Autodesk Fusion 360 part; units mm, degrees
(part 2 of 2)
sketch "Sketch9" plane through (0, 0, 0) normal (1, 0, 0) x (0, 1, 0)
  line L0 (195.5, 133.4393) -> (195.5, 130.2075)
  line L1 (208.5, 133) -> (208.5, 135.95)
  line L2 (196.5607, 125.5) -> (199.7925, 125.5)
  line L3 (190, 133.5) -> (190, 138.5)
  line L4 (190.5, 133) -> (190.5, 133.5)
  line L5 (205.95, 138.5) -> (205.95, 137.0107)
  line L6 (203.5, 140) -> (208.5, 140)
  line L7 (190, 126.5) -> (190.5, 126.5)
  line L8 (203.4393, 125.5) -> (200.2075, 125.5)
  line L9 (210, 126.5) -> (209.5, 126.5)
  line L10 (203.5, 120) -> (203.5, 120.5)
  line L11 (208.5, 124.05) -> (207.0107, 124.05)
  line L12 (192.9893, 124.05) -> (195.5, 126.5607)
  line L13 (190, 121.5) -> (190, 126.5)
  line L14 (209.5, 127) -> (208.5, 127)
  line L15 (194.05, 121.5) -> (194.05, 122.9893)
  line L16 (205.95, 137.0107) -> (203.4393, 134.5)
  line L17 (194.05, 138.5) -> (194.05, 137.0107)
  line L18 (191.5, 135.95) -> (192.9893, 135.95)
  line L19 (205.95, 121.5) -> (205.95, 122.9893)
  line L20 (197, 121.5) -> (194.05, 121.5)
  line L21 (209.5, 133.5) -> (209.5, 133)
  line L22 (209.5, 127) -> (209.5, 126.5)
  line L23 (208.5, 127) -> (208.5, 124.05)
  line L24 (197, 139.5) -> (197, 138.5)
  line L25 (203, 120.5) -> (203, 121.5)
  line L26 (196.5, 120) -> (191.5, 120)
  line L27 (196.5, 139.5) -> (197, 139.5)
  line L28 (210, 126.5) -> (210, 121.5)
  line L29 (204.5, 126.5607) -> (204.5, 129.7925)
  line L30 (205.95, 122.9893) -> (203.4393, 125.5)
  line L31 (208.5, 135.95) -> (207.0107, 135.95)
  line L32 (195.5, 126.5607) -> (195.5, 129.7925)
  line L33 (197, 120.5) -> (196.5, 120.5)
  line L34 (196.5, 140) -> (196.5, 139.5)
  line L35 (203, 139.5) -> (203.5, 139.5)
  line L36 (194.05, 137.0107) -> (196.5607, 134.5)
  line L37 (203, 139.5) -> (203, 138.5)
  line L38 (207.0107, 124.05) -> (204.5, 126.5607)
  line L39 (190, 133.5) -> (190.5, 133.5)
  line L40 (191.5, 140) -> (196.5, 140)
  line L41 (191.5, 127) -> (191.5, 124.05)
  line L42 (191.5, 124.05) -> (192.9893, 124.05)
  line L43 (203, 121.5) -> (205.95, 121.5)
  line L44 (190.5, 126.5) -> (190.5, 127)
  line L45 (196.5607, 134.5) -> (199.7925, 134.5)
  line L46 (203.5, 120.5) -> (203, 120.5)
  line L47 (203, 138.5) -> (205.95, 138.5)
  line L48 (192.9893, 135.95) -> (195.5, 133.4393)
  line L49 (203.5, 140) -> (203.5, 139.5)
  line L50 (210, 133.5) -> (209.5, 133.5)
  line L51 (197, 120.5) -> (197, 121.5)
  line L52 (196.5, 120) -> (196.5, 120.5)
  line L53 (191.5, 133) -> (191.5, 135.95)
  line L54 (194.05, 122.9893) -> (196.5607, 125.5)
  line L55 (209.5, 133) -> (208.5, 133)
  line L56 (190.5, 127) -> (191.5, 127)
  line L57 (210, 138.5) -> (210, 133.5)
  line L58 (207.0107, 135.95) -> (204.5, 133.4393)
  line L59 (190.5, 133) -> (191.5, 133)
  line L60 (208.5, 120) -> (203.5, 120)
  line L61 (197, 138.5) -> (194.05, 138.5)
  line L62 (203.4393, 134.5) -> (200.2075, 134.5)
  line L63 (204.5, 133.4393) -> (204.5, 130.2075)
  circle A0 centre (200, 130) radius 2.74
  arc A1 (210, 138.5) -> (208.5, 140) centre (208.5, 138.5) ccw
  arc A2 (199.7925, 134.5) -> (200.2075, 134.5) centre (200, 134.5) ccw
  arc A3 (208.5, 120) -> (210, 121.5) centre (208.5, 121.5) ccw
  arc A4 (204.5, 130.2075) -> (204.5, 129.7925) centre (204.5, 130) ccw
  arc A5 (191.5, 140) -> (190, 138.5) centre (191.5, 138.5) ccw
  arc A6 (190, 121.5) -> (191.5, 120) centre (191.5, 121.5) ccw
  arc A7 (195.5, 129.7925) -> (195.5, 130.2075) centre (195.5, 130) ccw
  arc A8 (200.2075, 125.5) -> (199.7925, 125.5) centre (200, 125.5) ccw
extrude "Extrude8" add sketch "Sketch9" along normal blind 300 separate body makes body 8
extrude "Extrude9" add sketch "Sketch8" along normal blind 80 separate body makes body 9 at (7.662, 198.5713, 93.3333) makes body 10 at (292.1841, 201.6544, 93.3333)
hidden bodies 5 6 8 9 10
named bodies: "2040 x-frame right", "2040 y-frame bottom", "2040 y-frame top", "2040 x-frame left", "2040 bridge-post left", "2040 bridge-post right", "2040 bridge", "2020 bridge", "2020 bride post left", "2020 bridge post right"
